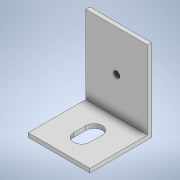
# Autodesk Inventor part: 規定課題1
Saved by Autodesk Inventor 2021 (Build 250183000, 183)
## iProperties
Created: 2021-09-20
Part Number: 規定課題1
Material: 一般
Document SubType Name: Modeling
Designer: ryusei
Density: 1 g/cm^3
Appearance: 既定
Author: ryusei
Autodesk Inventor part; units mm, degrees
ref_plane "YZ Plane" through (0, 0, 0) normal (1, 0, 0) x (0, 1, 0)
ref_plane "XZ Plane" through (0, 0, 0) normal (0, 1, 0) x (-1, 0, 0)
ref_plane "XY Plane" through (0, 0, 0) normal (0, 0, 1) x (1, 0, 0)
sketch "スケッチ1" plane through (0, 0, 0) normal (0, 0, 1) x (1, 0, 0)
  line L0 (0, 0) -> (30, 0)
  line L1 (30, 0) -> (30, 40)
  line L2 (30, 40) -> (0, 40)
  line L3 (0, 40) -> (0, 0)
  point P0 (15, 20)
  dimension "d0" = 30
  dimension "d1" = 40
  dimension "d2" = 20
  dimension "d3" = 15
  constraints: 8 end point, 2 parallel, 1 horizontal, 1 perpendicular
  measures "d0" distance between parallel lines of L1 L3
  measures "d1" distance between parallel lines of L0 L2
  measures "d2" distance from line of L2 point (15, 20)
  measures "d3" distance from line of L1 point (15, 20)
extrude "押し出し1" add sketch "スケッチ1" along normal blind 2
sketch "スケッチ2" plane through (0, 0, 2) normal (0, 0, 1) x (1, 0, 0)
  line L0 (30, 0) -> (30, 40) projected
  line L1 (30, 40) -> (0, 40) projected
  point P0 (0, 0)
  point P1 (15, 20)
  dimension "d6" = 15
  dimension "d7" = 20
  measures "d6" distance from line of L0 point (15, 20)
  measures "d7" distance from line of point (15, 20) L1
hole "穴1" at (15, 20, 2) direction (0, 0, -1) diameter 3.242 end through all thread size "M4x0.7" class "6H" standard "ISO Metric profile"
sketch "スケッチ5" plane through (0, 0, 2) normal (0, 0, 1) x (1, 0, 0)
  line L0 (0, 40) -> (0, 0) projected
  line L1 (0, 0) -> (30, 0) projected
  line L2 (0, 2) -> (30, 2)
  line L3 (30, 2) -> (30, 0)
  line L4 (30, 0) -> (0, 0)
  line L5 (0, 0) -> (0, 2)
  dimension "d15" = 2
  dimension "d16" = 30
  constraints: 8 end point, 2 parallel, 1 horizontal, 1 perpendicular, 1 point on line
  measures "d15" distance between parallel lines of L1 L2
  measures "d16" distance of L2.start L2.end
extrude "押し出し2" add sketch "スケッチ5" along normal blind 28
sketch "スケッチ10" plane through (0, 0, 0) normal (0, -1, 0) x (1, 0, 0)
  line L0 (11, 19) -> (19, 19)
  line L1 (19, 19) -> (19, 13)
  line L2 (19, 13) -> (11, 13)
  line L3 (11, 13) -> (11, 19)
  line L4 (30, 0) -> (30, 30) projected
  line L5 (0, 30) -> (30, 30) projected
  point P0 (0, 0)
  dimension "d32" = 8
  dimension "d33" = 11
  dimension "d34" = 11
  dimension "d35" = 6
  constraints: 8 end point, 2 parallel, 1 horizontal, 1 perpendicular
  measures "d32" distance between parallel lines of L3 L1
  measures "d33" distance between parallel lines of L4 L1
  measures "d34" distance between parallel lines of L0 L5
  measures "d35" distance between parallel lines of L2 L0
extrude "押し出し6" cut sketch "スケッチ10" against normal blind 10
sketch "スケッチ11" plane through (0, 0, 0) normal (0, -1, 0) x (1, 0, 0)
  line L0 (11, 19) -> (19, 19) projected
  circle A0 centre (15, 19) radius 4
  line L1 (11, 13) -> (19, 13) projected
  circle A1 centre (15, 13) radius 4
  point P0 (0, 0)
  point P1 (12.3542, 16)
  point P2 (17.6458, 16)
  constraints: 2 midpoint, 6 other
extrude "押し出し7" cut sketch "スケッチ11" against normal blind 10 contours A0 L0 | A0 A1 L1
sketch "スケッチ12" plane through (0, 0, 0) normal (0, -1, 0) x (1, 0, 0)
  line L0 (11, 13) -> (19, 13) projected
  circle A0 centre (15, 13) radius 4
  point P0 (0, 0)
  constraints: 1 midpoint, 3 other
extrude "押し出し8" cut sketch "スケッチ12" against normal blind 10 contours L0 A0 picked at (13.7054, 12.6809)
